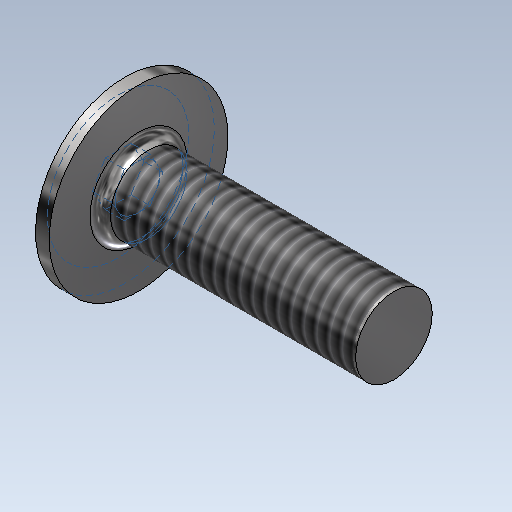
# Autodesk Inventor part: 超極低頭ネジL10
Saved by Autodesk Inventor 2020 (Build 240168000, 168)
## iProperties
Created: 2020-02-24
Part Number: 超極低頭ネジL10
Material: ステンレス鋼 440C
Catalog Web Link: www.cadenas.de
Description: CBSSE, CBSKE, CBSTSE-Ultra Low Head Cap Screws
Vendor: MISUMI
Document SubType Name: Modeling
Designer: psadmin
Manufacturer: MISUMI
Mass: 0.755034 g
Surface Area: 1.87243 cm^2
Volume: 0.0974238 cm^3
Density: 7.75 g/cm^3
Appearance: 半つや出し
Category: PARTsolutions
Company: MISUMI
PSOL_IDENT_0: {$CADENAS_DATA\23d-libs\misumi\metric\27_screws_nuts\cbsse.prj},179 {VTYP=3D},{NB=CBSKE3-6},{LINA=CB
PSOL_IDENT_1: SKE3-6},{NN=CBSSE, CBSKE, CBSTSE},{DATE=09.09.2019 15:27:56},{GEOMDATE=04.03.2010 00:00:00},{VERSION=
PSOL_IDENT_2: },{LINEID=30},{WBVAR=MAT,ST,L},{WBNUMERIC=L}  {NB=CBSKE3-6},{LINA=CBSKE3-6},{KT=DUMMY},{PN=CBSKE3-6}
PSOL_IDENT_3: ,{TYPE=CBSKE},{MAT=1},{MATA=  '1','Cold Forged Carbon Steel Wire SWCH12~18A','2','SUSXM7(30430 Stain
PSOL_IDENT_4: less Steel)'    },{HARD=HV400~},{ST=2},{STA=    '1', 'Nickel Plating', '2', 'Black Nickel Plating'
PSOL_IDENT_5: },{M=3},{M1=3.0},{L=6},{L0=6, 8, 10},{MP=3x0.5},{A=7},{E=0.8},{B=1.27},{C=1.75},{TT=0.75},{RR=0.
PSOL_IDENT_6: 4},{P=0.50}
NN: CBSSE, CBSKE, CBSTSE
NT: Ultra Low Head Cap Screws
NB: CBSKE3-6
NBSYN: $PN.
LINA: CBSKE3-6
PN: CBSKE3-6
MAT: Cold Forged Carbon Steel Wire SWCH12~18A
HARD: HV400~
ST: Black Nickel Plating
M: 3
L: 6
MP: 3x0.5
A: 7
E: 0.8
B: 1.27
C: 1.75
TT: 0.75
RR: 0.4
SUPPLIER: MISUMI
ARTICLENO: CBSKE3-6
BOMINFO: CBSKE3-6
CREATOR: CADENAS GmbH
Title: CBSKE3-6
Author: Cadenas PARTsolutions
Comments: Ultra Low Head Cap Screws
Autodesk Inventor part; units mm, degrees
ref_plane "YZ Plane" through (0, 0, 0) normal (1, 0, 0) x (0, 1, 0)
ref_plane "XZ Plane" through (0, 0, 0) normal (0, 1, 0) x (-1, 0, 0)
ref_plane "XY Plane" through (0, 0, 0) normal (0, 0, 1) x (1, 0, 0)
sketch "Sketch_1" plane through (0, 0, 0) normal (0, 0, 1) x (1, 0, 0)
  line L0 (6, 0) -> (0, 0)
  line L1 (-0.8, 0) -> (-0.8, 2.7673)
  line L2 (-0.8, 2.7673) -> (-0.5333, 3.5)
  line L3 (-0.5333, 3.5) -> (0, 3.5)
  line L4 (0, 3.5) -> (0, 1.9)
  arc A0 (0, 1.9) -> (0.4, 1.5) centre (0.4, 1.9) ccw
  line L5 (0.4, 1.5) -> (6, 1.5)
  line L6 (6, 1.5) -> (6, 0)
  line L7 (6, 0) -> (-0.8, 0)
  line L8 (0, 0) -> (-0.8, 0)
  dimension "d6" = 6
  constraints: 18 end point, 3 vertical, 2 point on circle, 2 point on line, 1 centre point, 5 other
  measures "d6" distance of L0.start L0.end
revolve "Revolution1" add sketch "Sketch_1" angle 360 about axis through (6, 0, 0) along (1, 0, 0)
sketch "Sketch_5" plane through (-0.05, 0, 0) normal (1, 0, 0) x (0, 0, -1)
  arc A0 (-0.6801, -0.1159) -> (-0.4404, -0.531) centre (-0.5499, -0.3175) ccw
  arc A1 (-0.341, -0.5357) -> (-0.4404, -0.531) centre (-0.3947, -0.62) ccw
  arc A2 (-0.341, -0.5357) -> (-0.2934, -0.5632) centre (0, 0) ccw
  arc A3 (-0.2397, -0.6469) -> (-0.2934, -0.5632) centre (-0.3396, -0.6519) ccw
  arc A4 (-0.2397, -0.6469) -> (0.2397, -0.6469) centre (0, -0.635) ccw
  arc A5 (0.2934, -0.5632) -> (0.2397, -0.6469) centre (0.3396, -0.6519) ccw
  arc A6 (0.2934, -0.5632) -> (0.341, -0.5357) centre (0, 0) ccw
  arc A7 (0.4404, -0.531) -> (0.341, -0.5357) centre (0.3947, -0.62) ccw
  arc A8 (0.4404, -0.531) -> (0.6801, -0.1159) centre (0.5499, -0.3175) ccw
  arc A9 (0.6344, -0.0275) -> (0.6801, -0.1159) centre (0.7343, -0.0318) ccw
  arc A10 (0.6344, -0.0275) -> (0.6344, 0.0275) centre (0, 0) ccw
  arc A11 (0.6801, 0.1159) -> (0.6344, 0.0275) centre (0.7343, 0.0318) ccw
  arc A12 (0.6801, 0.1159) -> (0.4404, 0.531) centre (0.5499, 0.3175) ccw
  arc A13 (0.341, 0.5357) -> (0.4404, 0.531) centre (0.3947, 0.62) ccw
  arc A14 (0.341, 0.5357) -> (0.2934, 0.5632) centre (0, 0) ccw
  arc A15 (0.2397, 0.6469) -> (0.2934, 0.5632) centre (0.3396, 0.6519) ccw
  arc A16 (0.2397, 0.6469) -> (-0.2397, 0.6469) centre (0, 0.635) ccw
  arc A17 (-0.2934, 0.5632) -> (-0.2397, 0.6469) centre (-0.3396, 0.6519) ccw
  arc A18 (-0.2934, 0.5632) -> (-0.341, 0.5357) centre (0, 0) ccw
  arc A19 (-0.4404, 0.531) -> (-0.341, 0.5357) centre (-0.3947, 0.62) ccw
  arc A20 (-0.4404, 0.531) -> (-0.6801, 0.1159) centre (-0.5499, 0.3175) ccw
  arc A21 (-0.6344, 0.0275) -> (-0.6801, 0.1159) centre (-0.7343, 0.0318) ccw
  arc A22 (-0.6344, 0.0275) -> (-0.6344, -0.0275) centre (0, 0) ccw
  arc A23 (-0.6801, -0.1159) -> (-0.6344, -0.0275) centre (-0.7343, -0.0318) ccw
  line L0 (0.5052, 0.875) -> (1.0104, 0)
  line L1 (1.0104, 0) -> (0.5052, -0.875)
  line L2 (0.5052, -0.875) -> (-0.5052, -0.875)
  line L3 (-0.5052, -0.875) -> (-1.0104, 0)
  line L4 (-1.0104, 0) -> (-0.5052, 0.875)
  line L5 (-0.5052, 0.875) -> (0.5052, 0.875)
  point P0 (0, 0.875)
  point P1 (0.7578, 0.4375)
  point P2 (-0.7578, 0.4375)
  point P3 (0, -0.875)
  point P4 (0.7578, -0.4375)
  point P5 (-0.7578, -0.4375)
  constraints: 49 point on circle, 24 centre point, 12 end point, 1 coincident, 1 midpoint, 13 other
extrude "Extrusion1" cut sketch "Sketch_5" against normal blind 0.75
sketch "Sketch_2" plane through (0, 0, 0) normal (0, 0, 1) x (1, 0, 0)
  line L0 (0.4552, 0) -> (0, 0)
  line L1 (-0.05, 0) -> (-0.05, 0.875)
  line L2 (-0.05, 0.875) -> (0.4552, 0)
  line L3 (0.4552, 0) -> (-0.05, 0)
  line L4 (-0.05, 0.875) -> (-0.8, 0.875) projected
  constraints: 8 end point, 1 point on line
revolve "Revolution2" cut sketch "Sketch_2" angle 360 about axis through (0.4552, 0, 0) along (1, 0, 0)
sketch "スケッチ4" plane through (6, 0, 0) normal (1, 0, 0) x (0, 0, -1)
  circle A0 centre (0, 0) radius 1.5 projected
extrude "押し出し2" add sketch "スケッチ4" along normal blind 4
thread "Thread1" size "M3x0.5" class "6g" standard "ANSI Metric M Profile" length 9.5 offset 0.1
body "Solid1"
